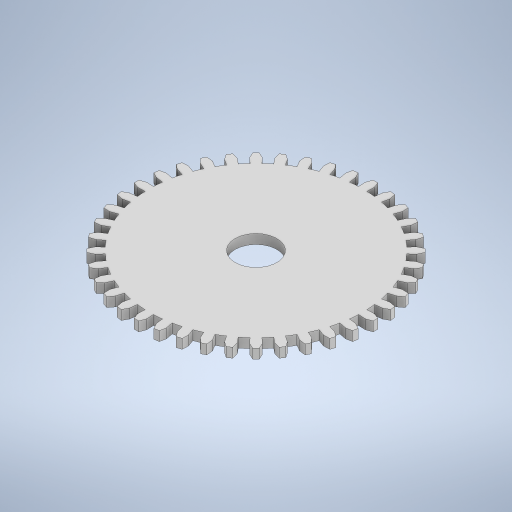
# Autodesk Inventor part: M3_45
Saved by Autodesk Inventor 2024.1 (Build 281209000, 209)
## iProperties
Created: 2024-04-01
Part Number: M3_45
Material: 一般
Document SubType Name: Modeling
Designer: hibik
Density: 1 g/cm^3
Appearance: 既定
Author: hibik
Autodesk Inventor part; units mm, degrees
ref_plane "YZ Plane" through (0, 0, 0) normal (1, 0, 0) x (0, 1, 0)
ref_plane "XZ Plane" through (0, 0, 0) normal (0, 1, 0) x (-1, 0, 0)
ref_plane "XY Plane" through (0, 0, 0) normal (0, 0, 1) x (1, 0, 0)
sketch "スケッチ1" plane through (0, 0, 0) normal (0, 1, 0) x (-1, 0, 0)
  circle A0 centre (0, 0) radius 60 construction
  circle A1 centre (0, 0) radius 63 construction
  line L0 (63, 1.2463) -> (63, -1.2463)
  line L1 (63, 1.2463) -> (59.9538, 2.355)
  line L2 (63, -1.2463) -> (59.9538, -2.355)
  line L3 (88.2, 0) -> (-88.2, 0) projected
  circle A2 centre (0, 0) radius 56.25
  line L4 (59.9538, -2.355) -> (56.2067, -2.2078)
  line L5 (59.9538, 2.355) -> (56.2067, 2.2078)
  line L6 (58.8472, 11.7048) -> (55.1693, 10.9733)
  line L7 (62.0294, 11.0863) -> (58.8472, 11.7048)
  line L8 (62.0294, 11.0863) -> (62.4193, 8.6245)
  line L9 (62.4193, 8.6245) -> (59.584, 7.0528)
  line L10 (59.584, 7.0528) -> (55.86, 6.612)
  line L11 (56.2917, 20.7665) -> (52.7735, 19.4686)
  line L12 (59.5314, 20.6533) -> (56.2917, 20.7665)
  line L13 (59.5314, 20.6533) -> (60.3017, 18.2828)
  line L14 (60.3017, 18.2828) -> (57.7472, 16.287)
  line L15 (57.7472, 16.287) -> (54.138, 15.2691)
  line L16 (52.35, 29.3168) -> (49.0782, 27.4845)
  line L17 (55.5676, 29.7118) -> (52.35, 29.3168)
  line L18 (55.5676, 29.7118) -> (56.6992, 27.491)
  line L19 (56.6992, 27.491) -> (54.4883, 25.1201)
  line L20 (54.4883, 25.1201) -> (51.0828, 23.5501)
  line L21 (47.1194, 37.1452) -> (44.1744, 34.8236)
  line L22 (50.2355, 38.0387) -> (47.1194, 37.1452)
  line L23 (50.2355, 38.0387) -> (51.7006, 36.0222)
  line L24 (51.7006, 36.0222) -> (49.8878, 33.3347)
  line L25 (49.8878, 33.3347) -> (46.7699, 31.2513)
  line L26 (40.7285, 44.059) -> (38.1829, 41.3053)
  line L27 (43.6665, 45.429) -> (40.7285, 44.059)
  line L28 (43.6665, 45.429) -> (45.429, 43.6665)
  line L29 (45.429, 43.6665) -> (44.059, 40.7285)
  line L30 (44.059, 40.7285) -> (41.3053, 38.1829)
  line L31 (33.3347, 49.8878) -> (31.2513, 46.7699)
  line L32 (36.0222, 51.7006) -> (33.3347, 49.8878)
  line L33 (36.0222, 51.7006) -> (38.0387, 50.2355)
  line L34 (38.0387, 50.2355) -> (37.1452, 47.1194)
  line L35 (37.1452, 47.1194) -> (34.8236, 44.1744)
  line L36 (25.1201, 54.4883) -> (23.5501, 51.0828)
  line L37 (27.491, 56.6992) -> (25.1201, 54.4883)
  line L38 (27.491, 56.6992) -> (29.7118, 55.5676)
  line L39 (29.7118, 55.5676) -> (29.3168, 52.35)
  line L40 (29.3168, 52.35) -> (27.4845, 49.0782)
  line L41 (16.287, 57.7472) -> (15.2691, 54.138)
  line L42 (18.2828, 60.3017) -> (16.287, 57.7472)
  line L43 (18.2828, 60.3017) -> (20.6533, 59.5314)
  line L44 (20.6533, 59.5314) -> (20.7665, 56.2917)
  line L45 (20.7665, 56.2917) -> (19.4686, 52.7735)
  line L46 (7.0528, 59.584) -> (6.612, 55.86)
  line L47 (8.6245, 62.4193) -> (7.0528, 59.584)
  line L48 (8.6245, 62.4193) -> (11.0863, 62.0294)
  line L49 (11.0863, 62.0294) -> (11.7048, 58.8472)
  line L50 (11.7048, 58.8472) -> (10.9733, 55.1693)
  line L51 (-2.355, 59.9538) -> (-2.2078, 56.2067)
  line L52 (-1.2463, 63) -> (-2.355, 59.9538)
  line L53 (-1.2463, 63) -> (1.2463, 63)
  line L54 (1.2463, 63) -> (2.355, 59.9538)
  line L55 (2.355, 59.9538) -> (2.2078, 56.2067)
  line L56 (-11.7048, 58.8472) -> (-10.9733, 55.1693)
  line L57 (-11.0863, 62.0294) -> (-11.7048, 58.8472)
  line L58 (-11.0863, 62.0294) -> (-8.6245, 62.4193)
  line L59 (-8.6245, 62.4193) -> (-7.0528, 59.584)
  line L60 (-7.0528, 59.584) -> (-6.612, 55.86)
  line L61 (-20.7665, 56.2917) -> (-19.4686, 52.7735)
  line L62 (-20.6533, 59.5314) -> (-20.7665, 56.2917)
  line L63 (-20.6533, 59.5314) -> (-18.2828, 60.3017)
  line L64 (-18.2828, 60.3017) -> (-16.287, 57.7472)
  line L65 (-16.287, 57.7472) -> (-15.2691, 54.138)
  line L66 (-29.3168, 52.35) -> (-27.4845, 49.0782)
  line L67 (-29.7118, 55.5676) -> (-29.3168, 52.35)
  line L68 (-29.7118, 55.5676) -> (-27.491, 56.6992)
  line L69 (-27.491, 56.6992) -> (-25.1201, 54.4883)
  line L70 (-25.1201, 54.4883) -> (-23.5501, 51.0828)
  line L71 (-37.1452, 47.1194) -> (-34.8236, 44.1744)
  line L72 (-38.0387, 50.2355) -> (-37.1452, 47.1194)
  line L73 (-38.0387, 50.2355) -> (-36.0222, 51.7006)
  line L74 (-36.0222, 51.7006) -> (-33.3347, 49.8878)
  line L75 (-33.3347, 49.8878) -> (-31.2513, 46.7699)
  line L76 (-44.059, 40.7285) -> (-41.3053, 38.1829)
  line L77 (-45.429, 43.6665) -> (-44.059, 40.7285)
  line L78 (-45.429, 43.6665) -> (-43.6665, 45.429)
  line L79 (-43.6665, 45.429) -> (-40.7285, 44.059)
  line L80 (-40.7285, 44.059) -> (-38.1829, 41.3053)
  line L81 (-49.8878, 33.3347) -> (-46.7699, 31.2513)
  line L82 (-51.7006, 36.0222) -> (-49.8878, 33.3347)
  line L83 (-51.7006, 36.0222) -> (-50.2355, 38.0387)
  line L84 (-50.2355, 38.0387) -> (-47.1194, 37.1452)
  line L85 (-47.1194, 37.1452) -> (-44.1744, 34.8236)
  line L86 (-54.4883, 25.1201) -> (-51.0828, 23.5501)
  line L87 (-56.6992, 27.491) -> (-54.4883, 25.1201)
  line L88 (-56.6992, 27.491) -> (-55.5676, 29.7118)
  line L89 (-55.5676, 29.7118) -> (-52.35, 29.3168)
  line L90 (-52.35, 29.3168) -> (-49.0782, 27.4845)
  line L91 (-57.7472, 16.287) -> (-54.138, 15.2691)
  line L92 (-60.3017, 18.2828) -> (-57.7472, 16.287)
  line L93 (-60.3017, 18.2828) -> (-59.5314, 20.6533)
  line L94 (-59.5314, 20.6533) -> (-56.2917, 20.7665)
  line L95 (-56.2917, 20.7665) -> (-52.7735, 19.4686)
  line L96 (-59.584, 7.0528) -> (-55.86, 6.612)
  line L97 (-62.4193, 8.6245) -> (-59.584, 7.0528)
  line L98 (-62.4193, 8.6245) -> (-62.0294, 11.0863)
  line L99 (-62.0294, 11.0863) -> (-58.8472, 11.7048)
  line L100 (-58.8472, 11.7048) -> (-55.1693, 10.9733)
  line L101 (-59.9538, -2.355) -> (-56.2067, -2.2078)
  line L102 (-63, -1.2463) -> (-59.9538, -2.355)
  line L103 (-63, -1.2463) -> (-63, 1.2463)
  line L104 (-63, 1.2463) -> (-59.9538, 2.355)
  line L105 (-59.9538, 2.355) -> (-56.2067, 2.2078)
  line L106 (-58.8472, -11.7048) -> (-55.1693, -10.9733)
  line L107 (-62.0294, -11.0863) -> (-58.8472, -11.7048)
  line L108 (-62.0294, -11.0863) -> (-62.4193, -8.6245)
  line L109 (-62.4193, -8.6245) -> (-59.584, -7.0528)
  line L110 (-59.584, -7.0528) -> (-55.86, -6.612)
  line L111 (-56.2917, -20.7665) -> (-52.7735, -19.4686)
  line L112 (-59.5314, -20.6533) -> (-56.2917, -20.7665)
  line L113 (-59.5314, -20.6533) -> (-60.3017, -18.2828)
  line L114 (-60.3017, -18.2828) -> (-57.7472, -16.287)
  line L115 (-57.7472, -16.287) -> (-54.138, -15.2691)
  line L116 (-52.35, -29.3168) -> (-49.0782, -27.4845)
  line L117 (-55.5676, -29.7118) -> (-52.35, -29.3168)
  line L118 (-55.5676, -29.7118) -> (-56.6992, -27.491)
  line L119 (-56.6992, -27.491) -> (-54.4883, -25.1201)
  line L120 (-54.4883, -25.1201) -> (-51.0828, -23.5501)
  line L121 (-47.1194, -37.1452) -> (-44.1744, -34.8236)
  line L122 (-50.2355, -38.0387) -> (-47.1194, -37.1452)
  line L123 (-50.2355, -38.0387) -> (-51.7006, -36.0222)
  line L124 (-51.7006, -36.0222) -> (-49.8878, -33.3347)
  line L125 (-49.8878, -33.3347) -> (-46.7699, -31.2513)
  line L126 (-40.7285, -44.059) -> (-38.1829, -41.3053)
  line L127 (-43.6665, -45.429) -> (-40.7285, -44.059)
  line L128 (-43.6665, -45.429) -> (-45.429, -43.6665)
  line L129 (-45.429, -43.6665) -> (-44.059, -40.7285)
  line L130 (-44.059, -40.7285) -> (-41.3053, -38.1829)
  line L131 (-33.3347, -49.8878) -> (-31.2513, -46.7699)
  line L132 (-36.0222, -51.7006) -> (-33.3347, -49.8878)
  line L133 (-36.0222, -51.7006) -> (-38.0387, -50.2355)
  line L134 (-38.0387, -50.2355) -> (-37.1452, -47.1194)
  line L135 (-37.1452, -47.1194) -> (-34.8236, -44.1744)
  line L136 (-25.1201, -54.4883) -> (-23.5501, -51.0828)
  line L137 (-27.491, -56.6992) -> (-25.1201, -54.4883)
  line L138 (-27.491, -56.6992) -> (-29.7118, -55.5676)
  line L139 (-29.7118, -55.5676) -> (-29.3168, -52.35)
  line L140 (-29.3168, -52.35) -> (-27.4845, -49.0782)
  line L141 (-16.287, -57.7472) -> (-15.2691, -54.138)
  line L142 (-18.2828, -60.3017) -> (-16.287, -57.7472)
  line L143 (-18.2828, -60.3017) -> (-20.6533, -59.5314)
  line L144 (-20.6533, -59.5314) -> (-20.7665, -56.2917)
  line L145 (-20.7665, -56.2917) -> (-19.4686, -52.7735)
  line L146 (-7.0528, -59.584) -> (-6.612, -55.86)
  line L147 (-8.6245, -62.4193) -> (-7.0528, -59.584)
  line L148 (-8.6245, -62.4193) -> (-11.0863, -62.0294)
  line L149 (-11.0863, -62.0294) -> (-11.7048, -58.8472)
  line L150 (-11.7048, -58.8472) -> (-10.9733, -55.1693)
  line L151 (2.355, -59.9538) -> (2.2078, -56.2067)
  line L152 (1.2463, -63) -> (2.355, -59.9538)
  line L153 (1.2463, -63) -> (-1.2463, -63)
  line L154 (-1.2463, -63) -> (-2.355, -59.9538)
  line L155 (-2.355, -59.9538) -> (-2.2078, -56.2067)
  line L156 (11.7048, -58.8472) -> (10.9733, -55.1693)
  line L157 (11.0863, -62.0294) -> (11.7048, -58.8472)
  line L158 (11.0863, -62.0294) -> (8.6245, -62.4193)
  line L159 (8.6245, -62.4193) -> (7.0528, -59.584)
  line L160 (7.0528, -59.584) -> (6.612, -55.86)
  line L161 (20.7665, -56.2917) -> (19.4686, -52.7735)
  line L162 (20.6533, -59.5314) -> (20.7665, -56.2917)
  line L163 (20.6533, -59.5314) -> (18.2828, -60.3017)
  line L164 (18.2828, -60.3017) -> (16.287, -57.7472)
  line L165 (16.287, -57.7472) -> (15.2691, -54.138)
  line L166 (29.3168, -52.35) -> (27.4845, -49.0782)
  line L167 (29.7118, -55.5676) -> (29.3168, -52.35)
  line L168 (29.7118, -55.5676) -> (27.491, -56.6992)
  line L169 (27.491, -56.6992) -> (25.1201, -54.4883)
  line L170 (25.1201, -54.4883) -> (23.5501, -51.0828)
  line L171 (37.1452, -47.1194) -> (34.8236, -44.1744)
  line L172 (38.0387, -50.2355) -> (37.1452, -47.1194)
  line L173 (38.0387, -50.2355) -> (36.0222, -51.7006)
  line L174 (36.0222, -51.7006) -> (33.3347, -49.8878)
  line L175 (33.3347, -49.8878) -> (31.2513, -46.7699)
  line L176 (44.059, -40.7285) -> (41.3053, -38.1829)
  line L177 (45.429, -43.6665) -> (44.059, -40.7285)
  line L178 (45.429, -43.6665) -> (43.6665, -45.429)
  line L179 (43.6665, -45.429) -> (40.7285, -44.059)
  line L180 (40.7285, -44.059) -> (38.1829, -41.3053)
  line L181 (49.8878, -33.3347) -> (46.7699, -31.2513)
  line L182 (51.7006, -36.0222) -> (49.8878, -33.3347)
  line L183 (51.7006, -36.0222) -> (50.2355, -38.0387)
  line L184 (50.2355, -38.0387) -> (47.1194, -37.1452)
  line L185 (47.1194, -37.1452) -> (44.1744, -34.8236)
  line L186 (54.4883, -25.1201) -> (51.0828, -23.5501)
  line L187 (56.6992, -27.491) -> (54.4883, -25.1201)
  line L188 (56.6992, -27.491) -> (55.5676, -29.7118)
  line L189 (55.5676, -29.7118) -> (52.35, -29.3168)
  line L190 (52.35, -29.3168) -> (49.0782, -27.4845)
  line L191 (57.7472, -16.287) -> (54.138, -15.2691)
  line L192 (60.3017, -18.2828) -> (57.7472, -16.287)
  line L193 (60.3017, -18.2828) -> (59.5314, -20.6533)
  line L194 (59.5314, -20.6533) -> (56.2917, -20.7665)
  line L195 (56.2917, -20.7665) -> (52.7735, -19.4686)
  line L196 (59.584, -7.0528) -> (55.86, -6.612)
  line L197 (62.4193, -8.6245) -> (59.584, -7.0528)
  line L198 (62.4193, -8.6245) -> (62.0294, -11.0863)
  line L199 (62.0294, -11.0863) -> (58.8472, -11.7048)
  line L200 (58.8472, -11.7048) -> (55.1693, -10.9733)
  circle A3 centre (0, 0) radius 11
  point P0 (63, 0)
  point P1 (62.2244, 9.8554)
  point P2 (59.9166, 19.4681)
  point P3 (56.1334, 28.6014)
  point P4 (50.9681, 37.0305)
  point P5 (44.5477, 44.5477)
  point P6 (37.0305, 50.9681)
  point P7 (28.6014, 56.1334)
  point P8 (19.4681, 59.9166)
  point P9 (9.8554, 62.2244)
  point P10 (0, 63)
  point P11 (-9.8554, 62.2244)
  point P12 (-19.4681, 59.9166)
  point P13 (-28.6014, 56.1334)
  point P14 (-37.0305, 50.9681)
  point P15 (-44.5477, 44.5477)
  point P16 (-50.9681, 37.0305)
  point P17 (-56.1334, 28.6014)
  point P18 (-59.9166, 19.4681)
  point P19 (-62.2244, 9.8554)
  point P20 (-63, 0)
  point P21 (-62.2244, -9.8554)
  point P22 (-59.9166, -19.4681)
  point P23 (-56.1334, -28.6014)
  point P24 (-50.9681, -37.0305)
  point P25 (-44.5477, -44.5477)
  point P26 (-37.0305, -50.9681)
  point P27 (-28.6014, -56.1334)
  point P28 (-19.4681, -59.9166)
  point P29 (-9.8554, -62.2244)
  point P30 (0, -63)
  point P31 (9.8554, -62.2244)
  point P32 (19.4681, -59.9166)
  point P33 (28.6014, -56.1334)
  point P34 (37.0305, -50.9681)
  point P35 (44.5477, -44.5477)
  point P36 (50.9681, -37.0305)
  point P37 (56.1334, -28.6014)
  point P38 (59.9166, -19.4681)
  point P39 (62.2244, -9.8554)
  point P40 (-51.0828, -23.5501)
  point P41 (-49.0782, -27.4845)
  point P42 (-46.7699, -31.2513)
  point P43 (-44.1744, -34.8236)
  point P44 (-34.8236, -44.1744)
  point P45 (-27.4845, -49.0782)
  point P46 (-19.4686, -52.7735)
  point P47 (-10.9733, -55.1693)
  point P48 (-6.612, -55.86)
  point P49 (2.2078, -56.2067)
  point P50 (6.612, -55.86)
  point P51 (10.9733, -55.1693)
  point P52 (15.2691, -54.138)
  point P53 (23.5501, -51.0828)
  point P54 (27.4845, -49.0782)
  point P55 (31.2513, -46.7699)
  point P56 (34.8236, -44.1744)
  point P57 (38.1829, -41.3053)
  point P58 (41.3053, -38.1829)
  point P59 (46.7699, -31.2513)
  point P60 (49.0782, -27.4845)
  point P61 (51.0828, -23.5501)
  point P62 (52.7735, -19.4686)
  point P63 (54.138, -15.2691)
  point P64 (55.1693, -10.9733)
  point P65 (55.86, 6.612)
  point P66 (55.1693, 10.9733)
  point P67 (52.7735, 19.4686)
  point P68 (49.0782, 27.4845)
  point P69 (46.7699, 31.2513)
  point P70 (44.1744, 34.8236)
  point P71 (41.3053, 38.1829)
  point P72 (38.1829, 41.3053)
  point P73 (34.8236, 44.1744)
  point P74 (31.2513, 46.7699)
  point P75 (27.4845, 49.0782)
  point P76 (23.5501, 51.0828)
  point P77 (19.4686, 52.7735)
  point P78 (15.2691, 54.138)
  point P79 (10.9733, 55.1693)
  point P80 (6.612, 55.86)
  point P81 (2.2078, 56.2067)
  point P82 (-2.2078, 56.2067)
  point P83 (-6.612, 55.86)
  point P84 (-10.9733, 55.1693)
  point P85 (-15.2691, 54.138)
  point P86 (-27.4845, 49.0782)
  point P87 (-31.2513, 46.7699)
  point P88 (-34.8236, 44.1744)
  point P89 (-38.1829, 41.3053)
  point P90 (-41.3053, 38.1829)
  point P91 (-44.1744, 34.8236)
  point P92 (-52.7735, 19.4686)
  point P93 (-54.138, 15.2691)
  point P94 (-55.1693, 10.9733)
  point P95 (-56.2067, 2.2078)
  point P96 (-56.2067, -2.2078)
  point P97 (-55.86, -6.612)
  point P98 (-55.1693, -10.9733)
  point P99 (-54.138, -15.2691)
  dimension "d5" = 112.5
  dimension "d0" = 120
  dimension "d1" = 126
  dimension "d3" = 20
  dimension "d4" = 20
  dimension "d14" = 4.71
  dimension "d18" = 360
  dimension "d23" = 22
  constraints: 400 end point, 81 point on line, 6 coincident, 3 centre point, 2 point on circle, 1 midpoint, 1 tangent, 1 vertical, 522 other
  measures "d0" diameter of A0
  measures "d1" diameter of A1
  measures "d3" angle of L3 L1
  measures "d4" angle of L3 L2
  measures "d14" distance of L2.end L1.end
  measures "d23" diameter of A3
extrude "押し出し1" add sketch "スケッチ1" along normal blind 5 contours L0 L3 A2 L5 L1 | L0 L2 L4 A2 L3 | A2 L3 A3 | L3 A3 A2 | A2 L6 L7 L8 L9 L10 | L196 L197 L198 L199 L200 A2 | A2 L101 L102 L103 L3 | L3 L103 L104 L105 A2 | A2 L11 L12 L13 L14 L15 | L191 L192 L193 L194 L195 A2 | L96 L97 L98 L99 L100 A2 | A2 L106 L107 L108 L109 L110 | A2 L16 L17 L18 L19 L20 | L186 L187 L188 L189 L190 A2 | L91 L92 L93 L94 L95 A2 | A2 L111 L112 L113 L114 L115 | A2 L21 L22 L23 L24 L25 | L181 L182 L183 L184 L185 A2 | L86 L87 L88 L89 L90 A2 | A2 L116 L117 L118 L119 L120 | A2 L26 L27 L28 L29 L30 | L176 L177 L178 L179 L180 A2 | L81 L82 L83 L84 L85 A2 | A2 L121 L122 L123 L124 L125 | A2 L31 L32 L33 L34 L35 | L171 L172 L173 L174 L175 A2 | L76 L77 L78 L79 L80 A2 | A2 L126 L127 L128 L129 L130 | A2 L36 L37 L38 L39 L40 | L166 L167 L168 L169 L170 A2 | L71 L72 L73 L74 L75 A2 | A2 L131 L132 L133 L134 L135 | A2 L41 L42 L43 L44 L45 | L161 L162 L163 L164 L165 A2 | L66 L67 L68 L69 L70 A2 | A2 L136 L137 L138 L139 L140 | A2 L46 L47 L48 L49 L50 | L156 L157 L158 L159 L160 A2 | L61 L62 L63 L64 L65 A2 | A2 L141 L142 L143 L144 L145 | A2 L51 L52 L53 L54 L55 | L151 L152 L153 L154 L155 A2 | L56 L57 L58 L59 L60 A2 | A2 L146 L147 L148 L149 L150
